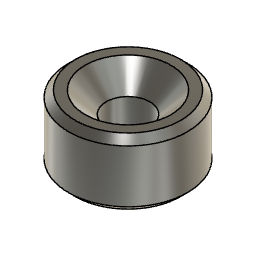
Load Pin (Autodesk Fusion 360 design; units mm, degrees)
Autodesk Fusion 360 part; units mm, degrees
sketch "Sketch1" plane through (0, 0, 0) normal (0, 0, 1) x (1, 0, 0)
  circle A0 centre (0, 0) radius 4.5
  circle A1 centre (0, 0) radius 1.5
  dimension "d1" = 9
  dimension "d4" = 3
  constraint coincident A0.centre A1.centre
  measures "d1" diameter of A0
  measures "d4" diameter of A1
extrude "Extrude1" add sketch "Sketch1" along normal blind 5
hole "Hole1" at (0, 0, 5) direction (0, 0, -1) diameter 3.3 depth 10 tip angle 118 countersink diameter 6.5 countersink angle 90
chamfer "Chamfer1" distance 0.5 angle 45 2 edges at (-4.1955, -1.6273, 5) (-4.1955, -1.6273, 0)
